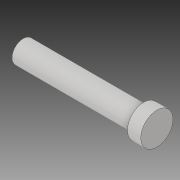
# Autodesk Inventor part: pin
Saved by Autodesk Inventor 2017 (Build 210142000, 142)
## iProperties
Created: 2021-04-21
Part Number: pin
Material: Generic
Document SubType Name: Modeling
Designer: Anthony
Density: 1 g/cm^3
Appearance: Default
Author: Anthony
Autodesk Inventor part; units mm, degrees
ref_plane "YZ Plane" through (0, 0, 0) normal (1, 0, 0) x (0, 1, 0)
ref_plane "XZ Plane" through (0, 0, 0) normal (0, 1, 0) x (-1, 0, 0)
ref_plane "XY Plane" through (0, 0, 0) normal (0, 0, 1) x (1, 0, 0)
sketch "Sketch1" plane through (0, 0, 0) normal (1, 0, 0) x (0, 1, 0)
  circle A0 centre (0, 0) radius 4.15
  dimension "d0" = 8.3
  constraints: 1 centre point, 1 coincident
  measures "d0" diameter of A0
extrude "Extrusion1" add sketch "Sketch1" along normal blind 40
sketch "Sketch2" plane through (40, 0, 0) normal (1, 0, 0) x (0, 0, -1)
  circle A0 centre (0, 0) radius 6
  constraints: 1 centre point, 1 coincident
extrude "Extrusion2" add sketch "Sketch2" against normal blind 5
thicken "Thicken1" operation add thickness 10 both sides no extend neighbours yes toward (-1, 0, 0) faces at (0, 1.0354, 0.9173)
body "Solid1"
